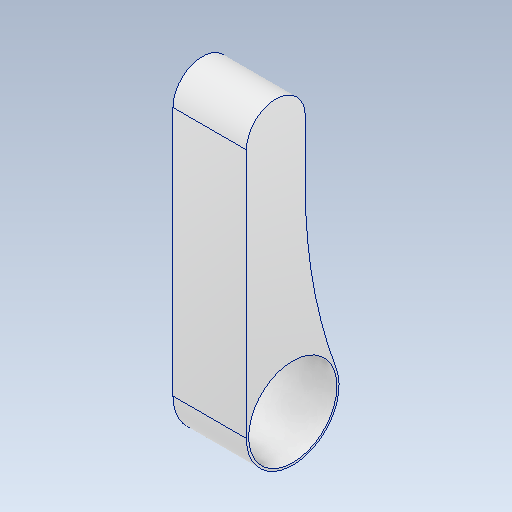
# Autodesk Inventor part: Strap connector thing (1)
Saved by Autodesk Inventor 2020 (Build 240168000, 168)
## iProperties
Created: 2020-05-08
Part Number: Strap connector thing (1)
Material: Aluminum 6061
Document SubType Name: Modeling
Designer: harry
Density: 2.7 g/cm^3
Appearance: Aluminum - Flat
Author: harry
Autodesk Inventor part; units mm, degrees
ref_plane "YZ Plane" through (0, 0, 0) normal (1, 0, 0) x (0, 1, 0)
ref_plane "XZ Plane" through (0, 0, 0) normal (0, 1, 0) x (-1, 0, 0)
ref_plane "XY Plane" through (0, 0, 0) normal (0, 0, 1) x (1, 0, 0)
sketch "Sketch1" plane through (0, 0, 0) normal (1, 0, 0) x (0, 1, 0)
  arc A0 (0, 1.575) -> (0.5456, -1.4775) centre (0, 0) ccw
  line L0 (0, 1.575) -> (8.5, 1.575)
  arc A1 (8.5, -0.425) -> (8.5, 1.575) centre (8.5, 0.575) ccw
  line L1 (8.5, -0.425) -> (6.4343, -0.425)
  arc A2 (6.4343, -0.425) -> (0.5456, -1.4775) centre (6.4343, -17.425) ccw
  dimension "d0" = 3.15
  dimension "d1" = 1
  dimension "d2" = 8.5
  dimension "d4" = 17
  dimension "d5" = 0.575
  constraints: 6 point on circle, 4 end point, 4 tangent, 3 centre point, 2 horizontal, 1 coincident
  measures "d0" diameter of A0
  measures "d1" radius of A1
  measures "d2" horizontal distance of point (0, 0) A1.centre
  measures "d4" radius of A2
  measures "d5" vertical distance of point (0, 0) A1.centre
extrude "Extrusion1" add sketch "Sketch1" along normal mid plane 2.5
sketch "Sketch2" plane through (1.25, 0, 0) normal (1, 0, 0) x (0, 0, -1)
  arc A0 (-1.575, 0) -> (1.4775, 0.5456) centre (0, 0) ccw projected
  constraints: 1 coincident
hole "Hole1" at (1.25, 0, 0) direction (-1, 0, 0) diameter 3 end through all
body "Solid1"
